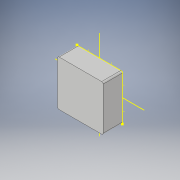
# Autodesk Inventor part: Glass
Saved by Autodesk Inventor 2019 (Build 230136000, 136)
## iProperties
Created: 2018-04-27
Part Number: Glass
Material: Generic
Document SubType Name: Modeling
Designer: Fierl
Density: 1 g/cm^3
Appearance: Default
Author: Fierl
Autodesk Inventor part; units mm, degrees
ref_plane "YZ Plane" through (0, 0, 0) normal (1, 0, 0) x (0, 1, 0)
ref_plane "XZ Plane" through (0, 0, 0) normal (0, 1, 0) x (-1, 0, 0)
ref_plane "XY Plane" through (0, 0, 0) normal (0, 0, 1) x (1, 0, 0)
sketch "Sketch3" plane through (0, 0, 0) normal (0, 0, -1) x (-1, 0, 0)
  line L0 (28, -30) -> (-28, -30)
  line L1 (-30, -28) -> (-30, 28)
  line L2 (-28, 30) -> (28, 30)
  line L3 (30, 28) -> (30, -28)
  circle A0 centre (0, 0) radius 23.5
  arc A1 (28, -30) -> (30, -28) centre (28, -28) ccw
  arc A2 (30, 28) -> (28, 30) centre (28, 28) ccw
  arc A3 (-30, -28) -> (-28, -30) centre (-28, -28) ccw
  arc A4 (-28, 30) -> (-30, 28) centre (-28, 28) ccw
  line L4 (0, -58.6799) -> (0, 58.6799)
  line L5 (58.6799, 0) -> (-58.6799, 0)
  point P0 (30, -30)
  point P1 (-30, -30)
  point P2 (30, 30)
  point P3 (26.5, 15)
  point P4 (26.5, 15)
  point P5 (22.4506, 22.4506)
  point P6 (-22.4506, 22.4506)
  point P7 (-22.4506, -22.4506)
  point P8 (22.4506, -22.4506)
  point P9 (15, 26.5)
  point P10 (-15, 26.5)
  point P11 (-26.5, -15)
  point P12 (15, -26.5)
  point P13 (-26.5, 15)
  point P14 (-15, -26.5)
  point P15 (26.5, -15)
sketch "Sketch2" plane through (0, 0, 0) normal (0, 0, 1) x (1, 0, 0)
  line L0 (28, 30) -> (-28, 30) projected
  arc A0 (-28, 30) -> (-30, 28) centre (-28, 28) ccw projected
  line L1 (-30, 28) -> (-30, -28) projected
  line L2 (30, -28) -> (30, 28) projected
  arc A1 (30, 28) -> (28, 30) centre (28, 28) ccw projected
  arc A2 (28, -30) -> (30, -28) centre (28, -28) ccw projected
  line L3 (-28, -30) -> (28, -30) projected
  arc A3 (-30, -28) -> (-28, -30) centre (-28, -28) ccw projected
  line L4 (-30, 30) -> (30, 30)
  line L5 (30, 30) -> (30, -30)
  line L6 (30, -30) -> (-30, -30)
  line L7 (-30, -30) -> (-30, 30)
  point P0 (0, 0)
  point P1 (-26.5, 15)
  point P2 (-22.4506, 22.4506)
  point P3 (-15, 26.5)
  point P4 (15, 26.5)
  point P5 (-26.5, -15)
  point P6 (-22.4506, -22.4506)
  point P7 (-15, -26.5)
  point P8 (15, -26.5)
  point P9 (22.4506, -22.4506)
  point P10 (26.5, -15)
  constraints: 8 end point, 2 parallel, 1 horizontal, 1 perpendicular
extrude "Extrusion2" add sketch "Sketch2" along normal blind 25.4 contours A1 L2 A2 L3 A3 L1 A0 L0
body "Solid1"
